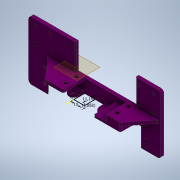
# Autodesk Inventor part: vydacha_4
Saved by Autodesk Inventor 2020 (Build 240168000, 168)
## iProperties
Created: 2022-07-27
Part Number: vydacha_4
Material: Типовые
Document SubType Name: ЛистМат
Designer: akapu
Density: 1 g/cm^3
Appearance: По умолчанию
Sheet Metal Rule: По умолчанию
Author: akapu
Autodesk Inventor part; units mm, degrees
ref_plane "YZ Plane" through (0, 0, 0) normal (1, 0, 0) x (0, 1, 0)
ref_plane "XZ Plane" through (0, 0, 0) normal (0, 1, 0) x (-1, 0, 0)
ref_plane "XY Plane" through (0, 0, 0) normal (0, 0, 1) x (1, 0, 0)
sketch "Эскиз1" plane through (0, 0, 0) normal (0, 0, 1) x (1, 0, 0)
  circle A0 centre (0, 0) radius 1.6
  line L0 (0, 0) -> (0, 14)
  line L1 (0, 14) -> (0, 28)
  line L2 (0, 28) -> (0, 44)
  line L3 (0, 28) -> (6, 28)
  line L4 (6, 28) -> (6, 44)
  line L5 (6, 44) -> (0, 44)
  line L6 (0, 44) -> (-8, 44)
  line L7 (-8, 44) -> (-8, 28)
  line L8 (-8, 28) -> (0, 28)
  circle A1 centre (0, 14) radius 1.6
  circle A2 centre (6, 28) radius 1.6
  circle A3 centre (6, 44) radius 1.6
  circle A4 centre (-8, 44) radius 1.6
  circle A5 centre (-8, 28) radius 1.6
  line L9 (0, 0) -> (96, 0)
  line L10 (96, 0) -> (96, 12.4)
  line L11 (96, 12.4) -> (96, 28)
  line L12 (96, 28) -> (96, 44)
  line L13 (96, 44) -> (90, 44)
  line L14 (90, 44) -> (90, 28)
  line L15 (90, 28) -> (96, 28)
  line L16 (96, 28) -> (104, 28)
  line L17 (104, 28) -> (104, 44)
  line L18 (104, 44) -> (96, 44)
  circle A6 centre (90, 44) radius 1.6
  circle A7 centre (90, 28) radius 1.6
  circle A8 centre (104, 28) radius 1.6
  circle A9 centre (104, 44) radius 1.6
  circle A10 centre (96, 12.4) radius 1.6
  circle A11 centre (96, 0) radius 1.6
  line L19 (48, 0) -> (83, 0)
  line L20 (0, 0) -> (0, -7)
  line L21 (0, -7) -> (10, -7)
  line L22 (96, -7) -> (96, 0)
  line L23 (83, -4) -> (83, 21)
  line L24 (83, 21) -> (13, 21)
  line L25 (13, 21) -> (13, -4)
  arc A12 (10, -7) -> (13, -4) centre (10, -4) ccw
  line L26 (96, -7) -> (86, -7)
  arc A13 (83, -4) -> (86, -7) centre (86, -4) ccw
  line L27 (0, 0) -> (-15, 0)
  line L28 (-15, 0) -> (-15, -4)
  line L29 (-12, -7) -> (0, -7)
  line L30 (96, 0) -> (111, 0)
  line L31 (111, 0) -> (111, -4)
  line L32 (108, -7) -> (96, -7)
  arc A14 (-15, -4) -> (-12, -7) centre (-12, -4) ccw
  arc A15 (108, -7) -> (111, -4) centre (108, -4) ccw
  line L33 (83, 21) -> (83, 49)
  line L34 (83, 49) -> (-12, 49)
  line L35 (-15, 46) -> (-15, 0)
  line L36 (83, 49) -> (108, 49)
  line L37 (111, 46) -> (111, 0)
  arc A16 (-12, 49) -> (-15, 46) centre (-12, 46) ccw
  arc A17 (111, 46) -> (108, 49) centre (108, 46) ccw
  point P0 (83, -7)
  point P1 (111, -7)
  point P2 (111, 49)
  dimension "d0" = 3.2
  dimension "d1" = 14
  dimension "d2" = 14
  dimension "d3" = 16
  dimension "d4" = 6
  dimension "d5" = 8
  dimension "d6" = 3.2
  dimension "d7" = 3.2
  dimension "d8" = 3.2
  dimension "d9" = 3.2
  dimension "d10" = 3.2
  dimension "d11" = 96
  dimension "d12" = 6
  dimension "d13" = 8
  dimension "d14" = 3.2
  dimension "d15" = 3.2
  dimension "d16" = 3.2
  dimension "d17" = 3.2
  dimension "d18" = 3.2
  dimension "d19" = 3.2
  dimension "d20" = 35
  dimension "d21" = 7
  dimension "d22" = 28
  dimension "d23" = 70
  dimension "d24" = 3
  dimension "d25" = 3
  dimension "d26" = 15
  dimension "d27" = 15
  dimension "d28" = 3
  dimension "d29" = 28
  dimension "d30" = 3
  constraints: 76 end point, 20 perpendicular, 19 point on line, 18 centre point, 12 coincident, 12 point on circle, 12 tangent, 5 vertical, 4 horizontal, 2 equal radius, 1 collinear, 1 midpoint
  measures "d0" diameter of A0
  measures "d1" distance of L0.start L0.end
  measures "d2" distance of L0.end L1.end
  measures "d3" distance of L1.end L2.end
  measures "d4" distance of L1.end L3.end
  measures "d5" distance of L2.end L6.end
  measures "d6" diameter of A1
  measures "d7" diameter of A2
  measures "d8" diameter of A3
  measures "d9" diameter of A4
  measures "d10" diameter of A5
  measures "d11" distance of L0.start L9.end
  measures "d12" distance of L12.end L13.end
  measures "d13" distance of L11.end L16.end
  measures "d14" diameter of A6
  measures "d15" diameter of A7
  measures "d16" diameter of A8
  measures "d17" diameter of A9
  measures "d18" diameter of A10
  measures "d19" diameter of A11
  measures "d20" distance of L19.start L19.end
  measures "d21" distance of L0.start L20.end
  measures "d22" distance of point (83, -7) L23.end
  measures "d23" distance of L23.end L24.end
  measures "d24" radius of A12
  measures "d25" radius of A13
  measures "d26" distance of L0.start L27.end
  measures "d27" distance of L22.end L30.end
  measures "d28" radius of A14
  measures "d29" distance of L23.end L33.end
  measures "d30" radius of A16
extrude "Выдавливание1" add sketch "Эскиз1" along normal blind 3 contours L9 L25 A12 L21 L20 A0 | A0 L27 L35 A16 L34 L33 L24 L25 L9 | L20 L29 A14 L28 L27 A0 | L23 L33 L36 A17 L37 L30 A11 L9 | L9 A11 L22 L26 A13 L23 | A11 L30 L31 A15 L32 L22 | A1 L1 L0 | L0 L1 A1 | L8 A5 L7 A4 L6 L2 | L2 L5 A3 L4 A2 L3 | A10 L11 L10 | L10 L11 A10 | L15 A7 L14 A6 L13 L12 | L12 L18 A9 L17 A8 L16
sketch "Эскиз9" plane through (0, 0, 3) normal (0, 0, 1) x (1, 0, 0)
  line L0 (-12, -7) -> (108, -7) projected
  line L1 (48, -7) -> (64.227, -7)
  line L2 (64.227, -7) -> (31.773, -7)
  line L3 (31.773, -7) -> (31.773, 4)
  line L4 (64.227, -7) -> (64.227, 4)
  circle A0 centre (31.773, 4) radius 1.6
  circle A1 centre (64.227, 4) radius 1.6
  point P0 (0, 0)
  dimension "d77" = 16.227
  dimension "d78" = 32.454
  dimension "d79" = 11
  dimension "d80" = 3.2
  dimension "d81" = 3.2
  constraints: 8 end point, 2 centre point, 2 coincident, 2 point on line, 1 midpoint, 1 perpendicular, 1 vertical
  measures "d77" distance of L1.start L1.end
  measures "d78" distance of L1.end L2.end
  measures "d79" distance of L2.end L3.end
  measures "d80" diameter of A0
  measures "d81" diameter of A1
extrude "Выдавливание7" cut sketch "Эскиз9" against normal blind 10
sketch "Эскиз10" plane through (0, 0, 3) normal (0, 0, 1) x (1, 0, 0)
  circle A0 centre (0, 0) radius 1.6 projected
  line L0 (0, 0) -> (4, 0)
  line L1 (4, 0) -> (4, -7)
  line L2 (-12, -7) -> (108, -7) projected
  line L3 (4, -7) -> (4, 7)
  circle A1 centre (96, 0) radius 1.6 projected
  line L4 (96, 0) -> (92, 0)
  line L5 (92, 0) -> (92, -7)
  line L6 (92, -7) -> (92, 7)
  line L7 (92, 7) -> (4, 7)
  line L8 (4, -7) -> (92, -7)
  line L9 (13, -4) -> (13, 21) projected
  line L10 (83, 21) -> (83, -4) projected
  line L11 (13, 10) -> (83, 10)
  line L12 (83, 10) -> (83, 21)
  line L13 (83, 21) -> (13, 21)
  line L14 (13, 21) -> (13, 10)
  line L15 (4, -7) -> (4, 9)
  line L16 (4, 9) -> (92, 9)
  line L17 (92, 9) -> (92, 7)
  line L18 (4, 9) -> (4, 11)
  line L19 (4, 11) -> (92, 11)
  line L20 (92, 11) -> (92, 9)
  point P0 (83, 11)
  point P1 (13, 11)
  dimension "d84" = 4
  dimension "d85" = 14
  dimension "d86" = 4
  dimension "d87" = 14
  dimension "d102" = 16
  dimension "d103" = 2
  constraints: 36 end point, 5 perpendicular, 5 point on line, 3 horizontal, 3 parallel, 2 collinear, 1 vertical
  measures "d84" distance of L0.start L0.end
  measures "d85" distance of L1.end L3.end
  measures "d86" distance of L4.start L4.end
  measures "d87" distance of L5.end L6.end
  measures "d102" distance of L1.end L15.end
  measures "d103" distance of L15.end L18.end
extrude "Выдавливание9" add sketch "Эскиз10" against normal blind 3 contours L9 L19 L10 L11 | L9 L13 L10 L19
extrude "Выдавливание8" cut sketch "Эскиз10" against normal blind 3 contours L3 L7 L6 L5 L2 L1 | L15 L16 L9 L7 | L9 L16 L10 L7 | L18 L19 L9 L16 | L10 L16 L17 L7 | L9 L11 L10 L16 | L10 L19 L20 L16 | L9 L19 L10 L11
sketch "Эскиз12" plane through (-12, -7, 0) normal (0, -1, 0) x (1, 0, 0)
  line L0 (120, 3) -> (0, 3) projected
  line L1 (120, 0) -> (0, 0) projected
  line L2 (0, 3) -> (120, 3) projected
  line L3 (16, 3) -> (15.6, 3)
  line L4 (12.2, 0) -> (12.7, 0)
  line L5 (10.4, 0) -> (13.6, 0) projected
  line L6 (16, 0) -> (16, 3) projected
  line L7 (16, 3) -> (16, 0)
  line L8 (16, 0) -> (12.7, 0)
  line L9 (12.7, 0) -> (12.9, 0)
  line L10 (10.4, 0) -> (13.6, 0) projected
  line L11 (12.9, 0) -> (15.6, 3)
  line L12 (106.4, 0) -> (109.6, 0) projected
  line L13 (108, 0) -> (107.1, 0)
  line L14 (16, 3) -> (104, 3) projected
  line L15 (104, 3) -> (104.4, 3)
  line L16 (104.4, 3) -> (107.1, 0)
  line L17 (104, 0) -> (16, 0) projected
  line L18 (107.1, 0) -> (104, 0)
  line L19 (104, 0) -> (104, 3)
  point P0 (12, 0)
  dimension "d99" = 0.4
  dimension "d100" = 0.5
  dimension "d101" = 0.2
  dimension "d104" = 0.9
  dimension "d105" = 0.4
  constraints: 22 end point, 4 point on line, 2 collinear, 2 perpendicular, 1 midpoint, 3 other
  measures "d99" distance of L3.start L3.end
  measures "d100" distance of L4.start L4.end
  measures "d101" distance of L8.end L9.end
  measures "d104" distance of L13.start L13.end
  measures "d105" distance of L14.end L15.end
extrude "Выдавливание11" cut sketch "Эскиз12" against normal up to surface (18 mm away) contours L16 L1 L19 L0 | L6 L1 L11 L0
sketch "Эскиз13" plane through (0, 0, 3) normal (0, 0, 1) x (1, 0, 0)
  circle A0 centre (0, 14) radius 1.6 projected
  circle A1 centre (0, 14) radius 1.6
  circle A2 centre (96, 14) radius 1.6
  point P0 (0, 0)
  dimension "d111" = 3.2
  constraints: 2 centre point, 1 coincident, 1 concentric
  measures "d111" diameter of A2
extrude "Выдавливание12" cut sketch "Эскиз13" against normal blind 10
sketch "Эскиз14" plane through (0, 0, 3) normal (0, 0, 1) x (1, 0, 0)
  line L0 (3.6, -7) -> (3.6, 11) projected
  line L1 (3.6, 11) -> (3.6, 16)
  line L2 (3.6, 16) -> (92.4, 16)
  line L3 (3.6, 11) -> (92.4, 11) projected
  line L4 (92.4, 16) -> (92.4, 11)
  line L5 (92.4, 11) -> (3.6, 11)
  line L6 (38, 16) -> (3.6, 16)
  line L7 (3.6, 24) -> (38, 24)
  line L8 (58, 16) -> (92.4, 16)
  line L9 (92.4, 16) -> (92.4, 24)
  line L10 (92.4, 24) -> (58, 24)
  line L11 (58, 24) -> (58, 16)
  line L12 (108, 24) -> (108, 21) projected
  line L13 (92.4, 24) -> (108, 24)
  line L14 (108, 24) -> (108, 21)
  line L15 (108, 21) -> (92.4, 21)
  line L16 (92.4, 21) -> (92.4, 24)
  line L17 (58, 16) -> (78.5, 16)
  line L18 (78.5, 16) -> (78.5, 18)
  line L19 (78.5, 18) -> (58, 18)
  line L20 (58, 18) -> (58, 16)
  line L21 (78.5, 18) -> (78.5, 24)
  line L22 (78.5, 29) -> (78.5, 21) projected
  line L23 (38, 24) -> (38, 31)
  line L24 (38, 24) -> (38, 21)
  line L25 (38, 21) -> (25, 21)
  line L26 (38, 34) -> (38, 31)
  line L27 (3.6, 34) -> (3.6, 31)
  line L28 (25, 21) -> (23.6154, 21)
  line L29 (23.6154, 21) -> (3.6, 21)
  line L30 (3.6, 21) -> (3.6, 24)
  line L31 (25, 30.5) -> (3.6, 30.5)
  line L32 (3.6, 30.5) -> (3.6, 33.5)
  line L33 (3.6, 33.5) -> (38, 33.5)
  line L34 (38, 33.5) -> (38, 30.5)
  line L35 (38, 30.5) -> (30, 30.5)
  line L36 (25, 30.5) -> (25, 24)
  line L37 (30, 30.5) -> (30, 24)
  point P0 (0, 0)
  point P1 (78.5, 23)
  point P2 (31, 24)
  dimension "d112" = 5
  dimension "d113" = 8
  dimension "d114" = 8
  dimension "d115" = 2
  dimension "d150" = 7
  dimension "d152" = 3
  dimension "d168" = 3
  dimension "d169" = 3
  constraints: 68 end point, 13 point on line, 9 equal length, 7 perpendicular, 4 horizontal, 3 vertical
  measures "d112" distance of L0.end L1.end
  measures "d113" distance of L6.end L7.start
  measures "d114" distance of L9.end L8.end
  measures "d115" distance of L18.end L17.end
  measures "d150" distance of L7.end L23.end
  measures "d152" distance of L7.end L24.end
  measures "d168" distance of L31.end L32.end
  measures "d169" distance of L33.end L34.end
extrude "Выдавливание13" add sketch "Эскиз14" along normal blind 20 contours L2 L18 L21 L10 L9 | L11 L19 L18 L2 | L9 L13 L12 L15 | L7 L24 L25 L28 L29 L30 | L36 L31 L32 L27 L33 L26 L23 L35 L37 L7
ref_plane "РабПлоскость1" through (31, 29, 3) normal (0, 1, 0) x (1, 0, 0)
sketch "Эскиз3" plane through (31, 29, 3) normal (0, 1, 0) x (1, 0, 0)
  line L0 (-18, 0) -> (0, 0) projected
  line L1 (0, 0) -> (2.55, 0)
  line L2 (0, 0) -> (7, 0) projected
  line L3 (2.55, 0) -> (2.55, -20)
  line L4 (0, -20) -> (7, -20) projected
  line L5 (54.5, 0) -> (54.5, -20) projected
  line L6 (54.5, 0) -> (51.95, 0)
  line L7 (77, 0) -> (-43, 0) projected
  line L8 (51.95, 0) -> (51.95, -20)
  line L9 (47.5, -20) -> (54.5, -20) projected
  line L10 (52, 3) -> (52, 0) projected
  line L11 (52, 0) -> (51.95, -4.7497)
  line L12 (51.95, -4.7497) -> (2.55, -4.7497)
  line L13 (2.55, -20) -> (2.55, -15.25)
  line L14 (2.55, -15.25) -> (51.95, -15.25)
  line L15 (51.95, -15.25) -> (51.95, -13.392)
  line L16 (51.95, -4.7497) -> (51.9696, -2.8918)
  line L17 (51.9696, -2.8918) -> (2.55, -2.8918)
  line L18 (51.95, -13.392) -> (2.55, -13.392)
  circle A0 centre (2.55, -13.392) radius 1.6
  circle A1 centre (2.55, -2.8918) radius 1.6
  circle A2 centre (51.9696, -2.8918) radius 1.6
  circle A3 centre (51.95, -13.392) radius 1.6
  point P0 (-31, 3)
  dimension "d43" = 2.55
  dimension "d44" = 2.55
  dimension "d45" = 4.75
  dimension "d46" = 4.75
  dimension "d179" = 1.858
  dimension "d180" = 1.858
  dimension "d181" = 3.2
  dimension "d182" = 3.2
  dimension "d183" = 3.2
  dimension "d184" = 3.2
  constraints: 24 end point, 12 point on line, 6 perpendicular, 4 centre point, 4 coincident
  measures "d43" distance of L0.end L1.end
  measures "d44" distance of L5.start L6.end
  measures "d45" distance of L10.end L11.end
  measures "d46" distance of L3.end L13.end
  measures "d179" distance of L14.end L15.end
  measures "d180" distance of L11.end L16.end
  measures "d181" diameter of A0
  measures "d182" diameter of A1
  measures "d183" diameter of A2
  measures "d184" diameter of A3
extrude "Выдавливание3" cut sketch "Эскиз3" against normal mid plane 40 contours A1 L17 L3 | L3 A1 | L17 A1 L3 | A2 L11 L17 L8 | L8 L17 A2 | L17 L8 A2 | A2 L11 | L17 L11 L8 | A0 L18 L3 | L3 A0 | L18 A0 L3 | A3 L8 | L8 L18 A3 | L18 L8 A3
sketch "Эскиз15" plane through (0, 0, 3) normal (0, 0, 1) x (1, 0, 0)
  line L0 (95.1, 11) -> (0.9, 11) projected
  line L1 (48, 11) -> (64.227, 11)
  line L2 (64.227, 11) -> (31.773, 11)
  line L3 (31.773, 11) -> (25.773, 11)
  line L4 (25.773, 11) -> (37.773, 11)
  line L5 (37.773, 11) -> (37.773, 13)
  line L6 (37.773, 13) -> (25.773, 13)
  line L7 (25.773, 13) -> (25.773, 11)
  line L8 (64.227, 11) -> (70.227, 11)
  line L9 (70.227, 11) -> (58.227, 11)
  line L10 (58.227, 11) -> (58.227, 13)
  line L11 (58.227, 13) -> (70.227, 13)
  line L12 (70.227, 13) -> (70.227, 11)
  line L13 (64.227, 13) -> (61.227, 13)
  line L14 (61.227, 13) -> (67.227, 13)
  line L15 (58, 16) -> (92.4, 16) projected
  line L16 (67.227, 13) -> (70.227, 13)
  line L17 (70.227, 13) -> (70.227, 16)
  line L18 (70.227, 16) -> (67.227, 16)
  line L19 (67.227, 16) -> (67.227, 13)
  line L20 (58.227, 13) -> (61.227, 13)
  line L21 (61.227, 13) -> (61.227, 16)
  line L22 (61.227, 16) -> (58.227, 16)
  line L23 (58.227, 16) -> (58.227, 13)
  line L24 (31.773, 13) -> (28.773, 13)
  line L25 (28.773, 13) -> (28.773, 16)
  line L26 (58, 16) -> (92.4, 16) projected
  line L27 (25.773, 13) -> (25.773, 16)
  line L28 (28.773, 16) -> (25.773, 16)
  line L29 (38, 21) -> (3.6, 21) projected
  line L30 (28.773, 16) -> (25.773, 16)
  line L31 (25.773, 16) -> (25.773, 21)
  line L32 (25.773, 21) -> (28.773, 21)
  line L33 (28.773, 21) -> (28.773, 16)
  point P0 (0, 0)
  point P1 (3.6, 16)
  point P2 (38, 16)
  dimension "d119" = 16.227
  dimension "d120" = 32.454
  dimension "d121" = 6
  dimension "d122" = 12
  dimension "d123" = 2
  dimension "d124" = 6
  dimension "d125" = 12
  dimension "d126" = 2
  dimension "d139" = 3
  dimension "d141" = 3
  constraints: 60 end point, 16 point on line, 9 perpendicular, 7 parallel, 3 horizontal, 3 midpoint
  measures "d119" distance of L1.start L1.end
  measures "d120" distance of L1.end L2.end
  measures "d121" distance of L2.end L3.end
  measures "d122" distance of L3.end L4.end
  measures "d123" distance of L4.end L5.end
  measures "d124" distance of L1.end L8.end
  measures "d125" distance of L8.end L9.end
  measures "d126" distance of L9.end L10.end
  measures "d139" distance of L13.start L13.end
  measures "d141" distance of L24.start L24.end
extrude "Выдавливание14" add sketch "Эскиз15" along normal blind 20 contours L0 L10 L11 L12 | L11 L19 L15 L17 | L23 L15 L21 L11 | L0 L7 L6 L5 | L27 L28 L25 L6 | L31 L29 L33 L28
sketch "Эскиз16" plane through (0.9, 11, 0) normal (0, -1, 0) x (1, 0, 0)
  line L0 (36.873, 23) -> (27.873, 23) projected
  line L1 (32.373, 23) -> (32.373, 0)
  line L2 (94.2, 0) -> (0, 0) projected
  line L3 (32.373, 0) -> (32.373, 8.243)
  line L4 (57.327, 23) -> (36.873, 23) projected
  line L5 (63.327, 23) -> (63.327, 0)
  line L6 (63.327, 0) -> (63.327, 8.243)
  circle A0 centre (32.373, 8.243) radius 1.7
  circle A1 centre (63.327, 8.243) radius 1.7
  circle A2 centre (63.327, 8.243) radius 6
  line L7 (57.327, 3) -> (57.327, 23) projected
  line L8 (69.327, 3) -> (69.327, 23) projected
  line L9 (57.327, 23) -> (69.327, 23)
  line L10 (69.327, 23) -> (69.327, 8.243)
  line L11 (69.327, 8.243) -> (57.327, 8.243)
  line L12 (57.327, 8.243) -> (57.327, 23)
  line L13 (36.873, 3) -> (36.873, 23) projected
  line L14 (24.873, 3) -> (24.873, 23) projected
  line L15 (36.873, 8.243) -> (24.873, 8.243)
  line L16 (24.873, 8.243) -> (24.873, 23)
  line L17 (24.873, 23) -> (36.873, 23)
  line L18 (36.873, 23) -> (36.873, 8.243)
  circle A3 centre (32.373, 8.243) radius 4.5
  point P0 (-0.9, 0)
  point P1 (57.327, 8.243)
  point P2 (27.873, 23)
  point P3 (34.073, 8.243)
  point P4 (30.673, 8.243)
  point P5 (27.873, 23)
  point P6 (27.873, 8.243)
  point P7 (36.873, 8.243)
  dimension "d129" = 8.243
  dimension "d130" = 8.243
  dimension "d131" = 3.4
  dimension "d132" = 3.4
  constraints: 24 end point, 7 point on line, 4 coincident, 4 parallel, 3 centre point, 3 perpendicular, 2 horizontal, 2 vertical, 1 midpoint, 1 tangent, 3 other
  measures "d129" distance of L1.end L3.end
  measures "d130" distance of L5.end L6.end
  measures "d131" diameter of A0
  measures "d132" diameter of A1
extrude "Выдавливание15" cut sketch "Эскиз16" against normal blind 5 contours L13 A3 L1 L0 | L1 A3 L15 L14 L17 L0 | L9 L5 A2 L7 | L9 L8 A2 L5 | L15 L1 A0 | A0 L1 L15 | L1 L15 A0 | L11 L5 A1 | A1 L5 L11 | A0 L15 L1 | A1 L11 L5 | L5 L11 A1
fillet "Сопряжение1" radius 0.7 2 edges at (61.227, 14.5, 13.4392) (67.227, 14.5, 13.4392)
sketch "Эскиз18" plane through (0, 0, 23) normal (0, 0, 1) x (1, 0, 0)
  line L0 (60.0383, 16) -> (61.227, 16) projected
  line L1 (58, 18) -> (78.5, 18) projected
  line L2 (61.227, 16) -> (67.227, 16)
  line L3 (67.227, 16) -> (67.227, 18)
  line L4 (67.227, 18) -> (61.227, 18)
  line L5 (61.227, 18) -> (61.227, 16)
  point P0 (0, 0)
  dimension "d142" = 6
  constraints: 8 end point, 2 parallel, 1 horizontal, 1 perpendicular, 1 point on line
  measures "d142" distance of L4.end L3.end
extrude "Выдавливание17" cut sketch "Эскиз18" against normal blind 20
fillet "Сопряжение2" radius 1 6 edges at (58, 17, 23) (61.227, 17, 23) (67.227, 17, 23) (78.5, 21, 23) (92.4, 18.5, 23) (108, 22.5, 23)
sketch "Эскиз19" plane through (58.227, 16, 3) normal (0, -1, 0) x (1, 0, 0)
  line L0 (-0.2688, 0) -> (3, 0)
  line L1 (3, 0) -> (3, 20.4543)
  line L2 (3, 20.4543) -> (-0.2688, 20.4543)
  line L3 (-0.2688, 20.4543) -> (-0.2688, 0)
  point P0 (-58.227, -3)
  constraints: 8 end point, 2 parallel, 1 horizontal, 1 perpendicular
extrude "Выдавливание18" cut sketch "Эскиз19" along normal blind 3 and the other way blind 10
sketch "Эскиз20" plane through (3.6, 21, 3) normal (0, -1, 0) x (1, 0, 0)
  circle A0 centre (29.95, 13.392) radius 1.6 projected
  line L0 (29.95, 13.392) -> (32.65, 13.392)
  line L1 (32.65, 13.392) -> (32.65, 2.8918)
  circle A1 centre (29.95, 2.8918) radius 1.6 projected
  line L2 (32.65, 2.8918) -> (29.95, 2.8918)
  circle A2 centre (79.35, 13.392) radius 1.6 projected
  line L3 (79.35, 13.392) -> (82.05, 13.392)
  line L4 (82.05, 13.392) -> (82.05, 2.8918)
  circle A3 centre (79.3696, 2.8918) radius 1.6 projected
  line L5 (82.05, 2.8918) -> (79.3696, 2.8918)
  line L6 (82.05, 11.8332) -> (79.35, 10.2743)
  line L7 (79.35, 10.2743) -> (76.65, 11.8332)
  line L8 (76.65, 11.8332) -> (76.65, 14.9508)
  line L9 (76.65, 14.9508) -> (79.35, 16.5097)
  line L10 (79.35, 16.5097) -> (82.05, 14.9508)
  line L11 (82.05, 14.9508) -> (82.05, 11.8332)
  line L12 (82.05, 1.3443) -> (79.3696, -0.2033)
  line L13 (79.3696, -0.2033) -> (76.6891, 1.3443)
  line L14 (76.6891, 1.3443) -> (76.6891, 4.4394)
  line L15 (76.6891, 4.4394) -> (79.3696, 5.9869)
  line L16 (79.3696, 5.9869) -> (82.05, 4.4394)
  line L17 (82.05, 4.4394) -> (82.05, 1.3443)
  line L18 (32.65, 1.333) -> (29.95, -0.2259)
  line L19 (29.95, -0.2259) -> (27.25, 1.333)
  line L20 (27.25, 1.333) -> (27.25, 4.4507)
  line L21 (27.25, 4.4507) -> (29.95, 6.0095)
  line L22 (29.95, 6.0095) -> (32.65, 4.4507)
  line L23 (32.65, 4.4507) -> (32.65, 1.333)
  line L24 (32.65, 11.8332) -> (29.95, 10.2743)
  line L25 (29.95, 10.2743) -> (27.25, 11.8332)
  line L26 (27.25, 11.8332) -> (27.25, 14.9508)
  line L27 (27.25, 14.9508) -> (29.95, 16.5097)
  line L28 (29.95, 16.5097) -> (32.65, 14.9508)
  line L29 (32.65, 14.9508) -> (32.65, 11.8332)
  point P0 (-3.6, -3)
  point P1 (29.95, 15.25)
  dimension "d185" = 2.7
  dimension "d186" = 2.7
  constraints: 60 end point, 4 coincident, 4 midpoint, 4 perpendicular, 2 horizontal, 52 other
  measures "d185" distance of L0.start L0.end
  measures "d186" distance of L3.start L3.end
extrude "Выдавливание19" cut sketch "Эскиз20" against normal blind 2 contours L1 L24 L25 L26 L27 L28 L29 | L1 L23 L18 L19 L20 L21 L22 | A1
sketch "Эскиз21" plane through (3.6, 21, 3) normal (0, -1, 0) x (1, 0, 0)
  line L0 (0, 20) -> (34.4, 20) projected
  line L1 (0, 0) -> (0, 20) projected
  line L2 (17.2, 20) -> (0, 0)
  line L3 (0, 0) -> (0, 20)
  line L4 (0, 20) -> (17.2, 20)
  point P0 (-3.6, -3)
  constraints: 6 end point, 1 midpoint, 1 perpendicular, 1 vertical
extrude "Выдавливание20" cut sketch "Эскиз21" against normal blind 20
sketch "Эскиз22" plane through (92.4, 21, 3) normal (0, -1, 0) x (1, 0, 0)
  arc A0 (0, 19) -> (-1, 20) centre (-1, 19) ccw projected
  line L0 (-1, 20) -> (0, 20)
  line L1 (15.6, 0) -> (0, 0) projected
  line L2 (0, 20) -> (15.6, 0)
  line L3 (15.6, 0) -> (15.6, 20)
  line L4 (15.6, 20) -> (0, 20)
  point P0 (-92.4, -3)
  constraints: 8 end point, 2 perpendicular, 1 horizontal, 1 point on line, 1 tangent
extrude "Выдавливание21" cut sketch "Эскиз22" against normal blind 20
fillet "Сопряжение3" radius 2 10 edges at (20.8, 22.5, 23) (20.8, 32, 23) (3.6, 22.5, 3) (3.6, 32, 3) (38, 22.5, 23) (92.4, 22.5, 23) (108, 22.5, 3) (30, 27.25, 23) (25, 27.25, 23) (38, 32, 23)
sketch "Эскиз23" plane through (0.9, 16, 0) normal (0, -1, 0) x (1, 0, 0)
  circle A0 centre (32.373, 8.243) radius 1.7 projected
  arc A1 (36.873, 8.243) -> (27.873, 8.243) centre (32.373, 8.243) ccw projected
  line L0 (67.327, 23) -> (90.5, 23) projected
  line L1 (24.873, 8.243) -> (24.873, 23)
  line L2 (24.873, 23) -> (27.8912, 23)
  line L3 (35.1, 23) -> (20.8179, 23) projected
  line L4 (27.873, 23) -> (27.873, 8.243) projected
  line L5 (27.873, 13.4392) -> (27.873, 23)
  line L6 (24.873, 3) -> (24.873, 23) projected
  line L7 (27.873, 8.243) -> (24.873, 3)
  line L8 (24.873, 8.243) -> (24.873, 23) projected
  line L9 (24.873, 3) -> (24.873, 23)
  line L10 (24.873, 23) -> (27.873, 23)
  line L11 (27.873, 23) -> (27.873, 8.243)
  point P0 (-0.9, 0)
  point P1 (27.1, 23)
  point P2 (27.873, 12.0377)
  point P3 (30.673, 8.243)
  point P4 (34.073, 8.243)
  point P5 (27.873, 23)
  constraints: 14 end point, 2 collinear, 2 perpendicular, 2 point on line, 1 vertical
extrude "Выдавливание22" cut sketch "Эскиз23" against normal mid plane 10 contours L1 L2 L4 L7 L6
fillet "Сопряжение4" radius 0.4 1 edges at (28.773, 17, 8.243)
sketch "Эскиз24" plane through (70.227, 16, 3) normal (0, -1, 0) x (1, 0, 0)
  circle A0 centre (12.723, 13.392) radius 1.6 projected
  line L0 (12.723, 13.392) -> (15.423, 13.392)
  line L1 (15.423, 13.392) -> (15.423, 2.8918)
  line L2 (15.423, 11.8332) -> (12.723, 10.2743)
  line L3 (12.723, 10.2743) -> (10.023, 11.8332)
  line L4 (10.023, 11.8332) -> (10.023, 14.9508)
  line L5 (10.023, 14.9508) -> (12.723, 16.5097)
  line L6 (12.723, 16.5097) -> (15.423, 14.9508)
  line L7 (15.423, 14.9508) -> (15.423, 11.8332)
  circle A1 centre (12.7426, 2.8918) radius 1.6 projected
  line L8 (15.423, 1.3443) -> (12.7426, -0.2033)
  line L9 (12.7426, -0.2033) -> (10.0621, 1.3443)
  line L10 (10.0621, 1.3443) -> (10.0621, 4.4394)
  line L11 (10.0621, 4.4394) -> (12.7426, 5.9869)
  line L12 (12.7426, 5.9869) -> (15.423, 4.4394)
  line L13 (15.423, 4.4394) -> (15.423, 1.3443)
  point P0 (-70.227, -3)
  point P1 (12.723, 15.25)
  point P2 (15.423, 11.8332)
  point P3 (15.423, 4.4394)
  dimension "d187" = 2.7
  constraints: 28 end point, 2 coincident, 2 midpoint, 1 horizontal, 1 perpendicular, 26 other
  measures "d187" distance of L0.start L0.end
extrude "Выдавливание23" cut sketch "Эскиз24" along normal blind 6 and the other way blind 3 contours A0 | L1 L2 L3 L4 L5 L6 L7 | L1 L13 L8 L9 L10 L11 L12 | A1
sketch "Эскиз25" plane through (0, 0, 23) normal (0, 0, 1) x (1, 0, 0)
  line L0 (2.6821, 24) -> (25, 24) projected
  line L1 (2.6821, 24) -> (38, 24)
  line L2 (38, 24) -> (38, 33.5)
  line L3 (38, 33.5) -> (2.6821, 33.5)
  line L4 (2.6821, 33.5) -> (2.6821, 24)
  point P0 (0, 0)
  constraints: 8 end point, 2 parallel, 1 horizontal, 1 perpendicular
extrude "Выдавливание24" cut sketch "Эскиз25" against normal up to surface (20 mm away)
sketch "Эскиз26" plane through (0.9, 11, 0) normal (0, -1, 0) x (1, 0, 0)
  line L0 (37.1, 3) -> (37.1, 21) projected
  line L1 (37.1, 3) -> (37.1, 13)
  line L2 (37.1, 13) -> (47.1, 13)
  line L3 (94.2, 0) -> (0, 0) projected
  line L4 (47.1, 0) -> (47.1, 11.142)
  line L5 (47.1, 11.142) -> (47.1, 13)
  point P0 (-0.9, 0)
  dimension "d175" = 10
  dimension "d176" = 10
  dimension "d177" = 11.142
  dimension "d178" = 1.858
  constraints: 8 end point, 1 horizontal, 1 midpoint, 1 point on line, 1 vertical
  measures "d175" distance of L0.start L1.end
  measures "d176" distance of L1.end L2.end
  measures "d177" distance of L4.start L4.end
  measures "d178" distance of L4.end L2.end
sketch "Эскиз27" plane through (0, 0, 3) normal (0, 0, 1) x (1, 0, 0)
  line L0 (31.95, 24) -> (35.15, 24) projected
  line L1 (33.55, 24) -> (29.55, 24)
  line L2 (29.55, 24) -> (29.55, 49)
  line L3 (108, 49) -> (-12, 49) projected
  line L4 (81.3696, 24) -> (84.5696, 24) projected
  line L5 (82.9696, 24) -> (86.9696, 24)
  line L6 (78.5, 24) -> (108.9765, 24) projected
  line L7 (86.9696, 24) -> (86.9696, 49)
  line L8 (86.9696, 49) -> (29.55, 49)
  line L9 (29.55, 24) -> (86.9696, 24)
  point P0 (0, 0)
  dimension "d190" = 4
  dimension "d191" = 4
  constraints: 12 end point, 3 perpendicular, 2 midpoint, 2 point on line, 1 collinear, 1 parallel
  measures "d190" distance of L1.start L1.end
  measures "d191" distance of L5.start L5.end
extrude "Выдавливание25" cut sketch "Эскиз27" against normal blind 6
fillet "Сопряжение5" radius 1 2 edges at (29.55, 36.5, 3) (86.9696, 36.5, 3)
equation "\"Радиус_гибки\" = Толщина"
equation "\"Ширина_просечки\" = Толщина"
equation "\"Глубина_просечки\" = 0.5 * Толщина"
equation "\"Размер_просечки\" = 4 * Толщина"
equation "\"Мин_остаток\" = 2 * Толщина"
equation "\"Радиус_перехода\" = Радиус_гибки"
equation "\"Радиус_Якоби\" = Толщина"
equation "\"Размер_зазора\" = Толщина"
equation "\"Толщина\" = 0.5"
